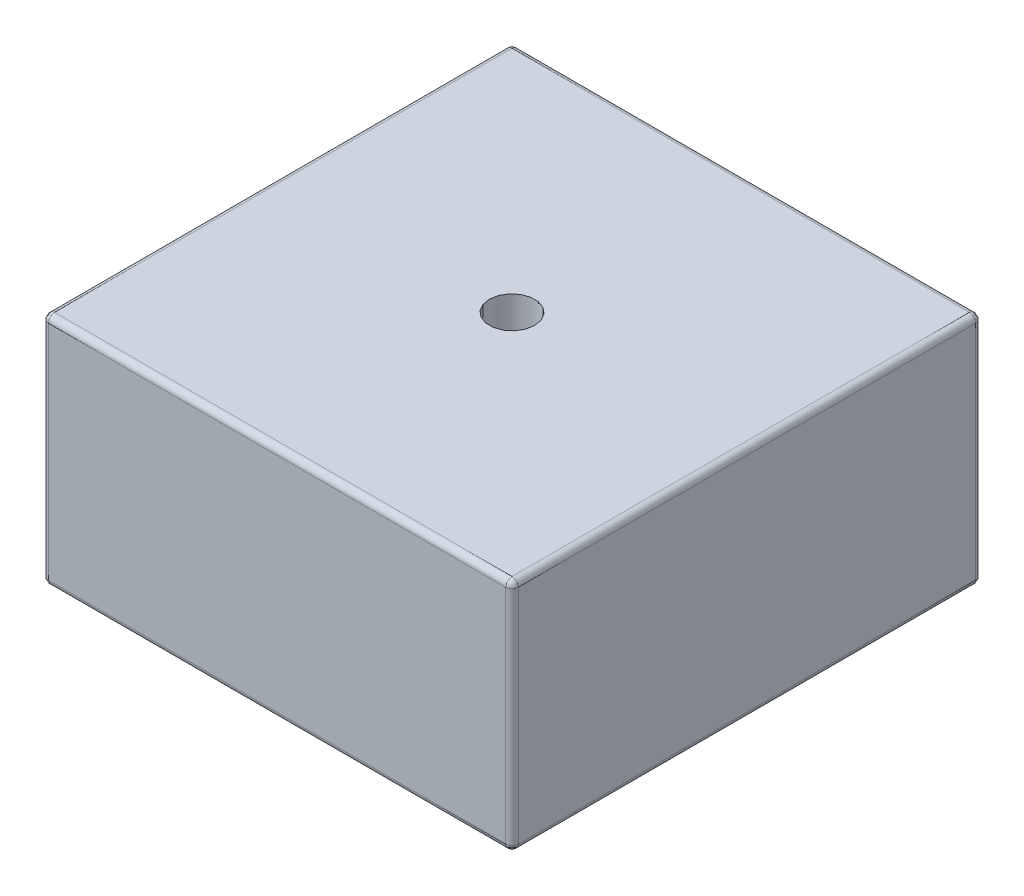
# Autodesk Inventor part: robotico
Saved by Autodesk Inventor 2016 (Build 200138000, 138)
## iProperties
Created: 2016-04-04
Part Number: robotico
Material: Genérico
Document SubType Name: Modeling
Designer: Usuario
Density: 1 g/cm^3
Appearance: Valor por defecto
Author: Usuario
Autodesk Inventor part; units mm, degrees
ref_plane "YZ Plane" through (0, 0, 0) normal (1, 0, 0) x (0, 1, 0)
ref_plane "XZ Plane" through (0, 0, 0) normal (0, 1, 0) x (-1, 0, 0)
ref_plane "XY Plane" through (0, 0, 0) normal (0, 0, 1) x (1, 0, 0)
sketch "Boceto1" plane through (0, 0, 0) normal (0, 1, 0) x (-1, 0, 0)
  line L0 (280, 9744) -> (430, 9744)
  line L1 (430, 9744) -> (430, 9594)
  line L2 (430, 9594) -> (280, 9594)
  line L3 (280, 9594) -> (280, 9744)
  point P0 (0, 0)
  dimension "d1" = 150
  dimension "d2" = 150
  dimension "d3" = 150
  constraints: 8 end point, 2 perpendicular, 1 horizontal
  measures "d1" distance of L0.start L0.end
  measures "d2" distance of L0.end L1.end
  measures "d3" distance of L1.end L2.end
extrude "Extrusión1" add sketch "Boceto1" along normal blind 75
sketch "Boceto2" plane through (0, 75, 0) normal (0, 1, 0) x (1, 0, 0)
  point P0 (0, 0)
sketch "Boceto3" plane through (0, 75, 0) normal (0, 1, 0) x (1, 0, 0)
  point P0 (0, 0)
sketch "Boceto4" plane through (0, 75, 0) normal (0, 1, 0) x (1, 0, 0)
  circle A0 centre (-355, -9669) radius 7.25
  point P0 (0, 0)
  point P1 (-430, -9744)
  dimension "d8" = 14.5
  constraints: 1 centre point
  measures "d8" diameter of A0
hole "Agujero1" at (-355, 75, 9669) direction (0, -1, 0) diameter 14.5 end through all
fillet "Empalme1" radius 2 12 edges at (-280, 75, 9669) (-280, 37.5, 9594) (-355, 75, 9594) (-430, 37.5, 9594) (-430, 75, 9669) (-355, 75, 9744) (-430, 37.5, 9744) (-280, 37.5, 9744) (-280, 0, 9669) (-355, 0, 9594) (-430, 0, 9669) (-355, 0, 9744)
